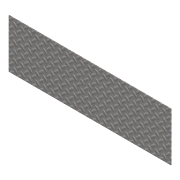
# Autodesk Inventor part: FE-00014-01
Saved by Autodesk Inventor 2012 (Build 160160000, 160)
## iProperties
Company: FIRST
Created: 2008-05-25
Part Number: FE-00014-01
Document SubType Name: Modeling
Designer: dfoster
Density: 1 g/cm^3
Description: Ramp Plate
Material: Default
Title: Ramp Plate
Author: dfoster
Autodesk Inventor part; units mm, degrees
ref_plane "YZ Plane" through (0, 0, 0) normal (1, 0, 0) x (0, 1, 0)
ref_plane "XZ Plane" through (0, 0, 0) normal (0, 1, 0) x (-1, 0, 0)
ref_plane "XY Plane" through (0, 0, 0) normal (0, 0, 1) x (1, 0, 0)
sketch "Sketch1" plane through (0, 0, 0) normal (0, 0, 1) x (1, 0, 0)
  line L0 (-26.9875, 22.225) -> (989.0125, 22.225)
  line L1 (989.0125, 22.225) -> (989.0125, -282.575)
  line L2 (989.0125, -282.575) -> (-26.9875, -282.575)
  line L3 (-26.9875, -282.575) -> (-26.9875, 22.225)
  dimension "d0" = 1016
  dimension "d1" = 304.8
  constraints: 8 end point, 2 parallel, 1 horizontal, 1 perpendicular
  measures "d0" distance of L0.start L0.end
  measures "d1" distance of L2.end L0.start
extrude "Extrusion1" add sketch "Sketch1" along normal blind 4.7625
body "Solid1"
